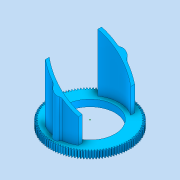
# Autodesk Inventor part: test_rotation
Saved by Autodesk Inventor 2022 (Build 260153000, 153)
## iProperties
Created: 2022-07-27
Part Number: test_rotation
Material: Générique
Document SubType Name: Modeling
Designer: andre
Density: 1 g/cm^3
Appearance: Par défaut(1)
Author: andre
Autodesk Inventor part; units mm, degrees
ref_plane "YZ Plane" through (0, 0, 0) normal (1, 0, 0) x (0, 1, 0)
ref_plane "XZ Plane" through (0, 0, 0) normal (0, 1, 0) x (-1, 0, 0)
sketch "Esquisse1" plane through (0, 0, 0) normal (0, 1, 0) x (-1, 0, 0)
  line L0 (16.5, -7.5) -> (-16.5, -7.5) construction
  line L1 (-16.5, -7.5) -> (-16.5, 7.5) construction
  line L2 (-16.5, 7.5) -> (16.5, 7.5) construction
  line L3 (16.5, 7.5) -> (16.5, -7.5) construction
  circle A0 centre (5, 0) radius 4.7 construction
  circle A1 centre (-5, 0) radius 5.2 construction
  circle A2 centre (0, -26.5) radius 17.5 construction
  line L4 (20.996, -26.9106) -> (-20.996, -26.0894) construction
  circle A3 centre (20.996, -26.9106) radius 2 construction
  circle A4 centre (-20.996, -26.0894) radius 2 construction
  arc A5 (23.507, -30.0242) -> (23.6268, -23.8975) centre (20.996, -26.9106) ccw construction
  arc A6 (-23.507, -22.9758) -> (-23.6268, -29.1025) centre (-20.996, -26.0894) ccw construction
  line L5 (-23.6268, -29.1025) -> (-11.5099, -39.6823) construction
  line L6 (-23.507, -22.9758) -> (-10.9858, -12.8779) construction
  line L7 (23.6268, -23.8975) -> (11.5099, -13.3177) construction
  line L8 (23.507, -30.0242) -> (10.9858, -40.1221) construction
  circle A7 centre (0, -26.5) radius 4 construction
  line L9 (5, 0) -> (-5, 0) construction
  line L10 (0, 0) -> (0, -26.5) construction
  circle A8 centre (0, 0) radius 10.5 construction
  circle A9 centre (0, 0) radius 22.5
  circle A10 centre (0, 0) radius 15.15
  point P0 (0, 0)
  point P1 (0, -9)
  point P2 (0, -22.5)
  dimension "d19" = 45
  dimension "d0" = 15
  dimension "d1" = 33
  dimension "d2" = 7.5
  dimension "d3" = 7.5
  dimension "d4" = 10
  dimension "d5" = 11.5
  dimension "d6" = 9.4
  dimension "d7" = 10.4
  dimension "d8" = 35
  dimension "d9" = 4
  dimension "d10" = 4
  dimension "d12" = 42
  dimension "d13" = 21
  dimension "d14" = 4
  dimension "d15" = 4
  dimension "d16" = 8
  dimension "d17" = 5
  dimension "d18" = 21
  dimension "d27" = 7.35
  constraints: 22 end point, 10 centre point, 9 point on circle, 8 coincident, 8 tangent, 4 midpoint, 2 parallel, 2 point on line, 1 horizontal, 1 perpendicular, 1 vertical, 1 vertical alignment, 3 other
  measures "d0" distance of L0.end L1.end
  measures "d1" distance of L1.end L2.end
  measures "d2" distance from line of L2 L9.start
  measures "d3" distance from line of L2 L9.end
  measures "d4" distance of L9.start L9.end
  measures "d5" distance from line of L3 L9.start
  measures "d6" diameter of A0
  measures "d7" diameter of A1
  measures "d8" diameter of A2
  measures "d9" diameter of A3
  measures "d10" diameter of A4
  measures "d12" distance of L4.start L4.end
  measures "d13" distance of L4.start A2.centre
  measures "d14" radius of A5
  measures "d15" radius of A6
  measures "d16" diameter of A7
  measures "d17" distance of L9.end point (0, 0)
  measures "d18" diameter of A8
extrude "Extrusion1" add sketch "Esquisse1" along normal blind 4
sketch "Esquisse2" plane through (0, 4, 0) normal (0, 1, 0) x (1, 0, 0)
  point P0 (0, 0)
sketch "Esquisse3" plane through (0, 4, 0) normal (0, 1, 0) x (1, 0, 0)
  line L0 (-22.4947, 0.4891) -> (-23.7228, 0.0662)
  line L1 (-22.4947, -0.4891) -> (-23.7228, -0.0662)
  circle A0 centre (0, 0) radius 22.5 projected
  arc A1 (-23.7228, 0.0662) -> (-23.7228, -0.0662) centre (-23.7, 0) ccw
  circle A2 centre (0, 0) radius 22.5 projected
  line L2 (-22.5, 0) -> (-28.4999, 0) construction
  line L3 (-45.1178, -23.4894) -> (-45.1178, 22.4675) construction
  line L4 (-45.1178, 22.4675) -> (-9.8799, 22.4675) construction
  line L5 (-9.8799, 22.4675) -> (-9.8799, -23.4894) construction
  line L6 (-9.8799, -23.4894) -> (-45.1178, -23.4894) construction
  circle A3 centre (-30.2354, 2.3473) radius 4 construction
  dimension "d30" = 0.07
  dimension "d31" = 1.2
  dimension "d32" = 19
  dimension "d33" = 19
  dimension "d66" = 8
  constraints: 6 end point, 5 point on circle, 2 centre point, 2 point on line, 2 tangent, 1 coincident, 1 horizontal, 2 other
  measures "d30" radius of A1
  measures "d31" distance of A1.centre L2.start
  measures "d32" angle of L0 L2
  measures "d33" angle of L2 L1
  measures "d66" diameter of A3
extrude "Extrusion2" add sketch "Esquisse3" against normal up to surface (4 mm away) contours A0 L1 A1 L0
pattern_circular "Réseau circulaire1" count 112 over 360 about axis through (0, 0, 0) along (0, 1, 0) of "Extrusion2"
sketch "Esquisse8" plane through (0, 4, 0) normal (0, 1, 0) x (1, 0, 0)
  line L0 (12.5, -12.5) -> (-12.5, -12.5) construction
  line L1 (-12.5, -12.5) -> (-12.5, 12.5) construction
  line L2 (-12.5, 12.5) -> (12.5, 12.5) construction
  line L3 (12.5, 12.5) -> (12.5, -12.5) construction
  line L4 (12.5, -12.5) -> (-12.5, 12.5) construction
  line L5 (-12.5, -12.5) -> (12.5, 12.5) construction
  circle A0 centre (0, 0) radius 17.15
  circle A1 centre (0, 0) radius 15.15 projected
  arc A2 (1.842, 20.529) -> (-1.842, 20.529) centre (0, 19.75) ccw
  line L6 (0, 0) -> (0, -7.2291)
  arc A3 (10, 14.665) -> (0, 17.75) centre (0, 0) ccw
  line L7 (10, 14.665) -> (10, 17.0312)
  arc A4 (10, 17.0312) -> (3.1578, 19.4959) centre (0, 0) ccw
  circle A5 centre (0, 0) radius 15.15 projected
  line L8 (0, 0) -> (-6.0663, 0)
  arc A6 (1.842, 20.529) -> (3.1578, 19.4959) centre (3.4342, 21.2024) ccw
  arc A7 (0, 17.75) -> (-10, 14.665) centre (0, 0) ccw
  line L9 (-10, 14.665) -> (-10, 17.0312)
  arc A8 (-3.1578, 19.4959) -> (-10, 17.0312) centre (0, 0) ccw
  arc A9 (-3.1578, 19.4959) -> (-1.842, 20.529) centre (-3.4342, 21.2024) ccw
  arc A10 (-1.842, -20.529) -> (1.842, -20.529) centre (0, -19.75) ccw
  arc A11 (0, -17.75) -> (10, -14.665) centre (0, 0) ccw
  line L10 (10, -14.665) -> (10, -17.0312)
  arc A12 (3.1578, -19.4959) -> (10, -17.0312) centre (0, 0) ccw
  arc A13 (3.1578, -19.4959) -> (1.842, -20.529) centre (3.4342, -21.2024) ccw
  arc A14 (-10, -17.0312) -> (-3.1578, -19.4959) centre (0, 0) ccw
  arc A15 (-1.842, -20.529) -> (-3.1578, -19.4959) centre (-3.4342, -21.2024) ccw
  arc A16 (-10, -14.665) -> (0, -17.75) centre (0, 0) ccw
  line L11 (-10, -14.665) -> (-10, -17.0312)
  dimension "d120" = 25
  dimension "d121" = 2
  dimension "d122" = 4
  dimension "d124" = 0.6
  dimension "d126" = 10
  dimension "d127" = 2
  dimension "d128" = 1.7288
  constraints: 28 point on circle, 24 end point, 17 symmetric about line, 15 centre point, 6 coincident, 3 tangent, 2 horizontal, 2 midpoint, 2 parallel, 2 perpendicular, 2 vertical, 1 point on line, 10 other
  measures "d120" distance of L0.end L1.end
  measures "d121" radial gap between concentric circles of A0 A1
  measures "d122" diameter of A2
  measures "d126" distance from line of L7 A2.centre
  measures "d127" radial gap between concentric circles of A4 A3
  measures "d128" radius of A6
extrude "Extrusion5" add sketch "Esquisse8" along normal blind 35 contours A6 A4 L7 A3 A7 L9 A8 A9 A2 | A15 A14 L11 A16 A11 L10 A12 A13 A10
ref_plane "Plan de construction2" through (-10, 39, 14.665) normal (-0.7071068, -0.7071068, 0) x (0, 0, 1)
sketch "Esquisse9" plane through (0, 39, 0) normal (0, 1, 0) x (1, 0, 0)
  arc A0 (-10, -17.0312) -> (-3.1578, -19.4959) centre (0, 0) ccw projected
  arc A1 (-1.842, -20.529) -> (-3.1578, -19.4959) centre (-3.4342, -21.2024) ccw projected
  arc A2 (-1.842, -20.529) -> (1.842, -20.529) centre (0, -19.75) ccw projected
  arc A3 (3.1578, -19.4959) -> (1.842, -20.529) centre (3.4342, -21.2024) ccw projected
  arc A4 (3.1578, -19.4959) -> (10, -17.0312) centre (0, 0) ccw projected
  line L0 (10, -17.0312) -> (10, -14.665) projected
  arc A5 (-10, -14.665) -> (10, -14.665) centre (0, 0) ccw projected
  line L1 (-10, -14.665) -> (-10, -17.0312) projected
  arc A6 (10, 17.0312) -> (3.1578, 19.4959) centre (0, 0) ccw projected
  arc A7 (1.842, 20.529) -> (3.1578, 19.4959) centre (3.4342, 21.2024) ccw projected
  arc A8 (1.842, 20.529) -> (-1.842, 20.529) centre (0, 19.75) ccw projected
  arc A9 (-3.1578, 19.4959) -> (-1.842, 20.529) centre (-3.4342, 21.2024) ccw projected
  arc A10 (-3.1578, 19.4959) -> (-10, 17.0312) centre (0, 0) ccw projected
  line L2 (-10, 17.0312) -> (-10, 14.665) projected
  arc A11 (10, 14.665) -> (-10, 14.665) centre (0, 0) ccw projected
  line L3 (10, 14.665) -> (10, 17.0312) projected
extrude "Extrusion6" cut sketch "Esquisse9" against normal up to surface surface through (-10, 39, 14.665) normal (-0.7071068, -0.7071068, 0)
equation "\"d5\" = -0.5 * d4 + 0.5 * d1"
equation "\"d13\" = 0.5 * d12"
equation "\"d17\" = 0.5 * d4"
